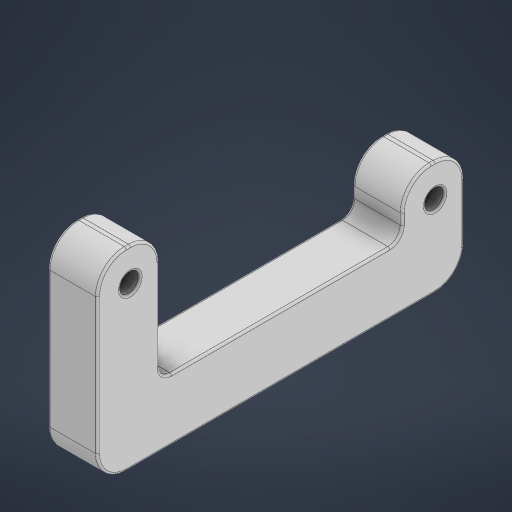
# Autodesk Inventor part: carb-holder
Saved by Autodesk Inventor 2024.2 (Build 282272000, 272)
## iProperties
Created: 2025-06-22
Part Number: carb-holder
Material: Generic
Document SubType Name: Modeling
Designer: Moe
Density: 1 g/cm^3
Appearance: Default
Author: Moe
Autodesk Inventor part; units mm, degrees
ref_plane "YZ Plane" through (0, 0, 0) normal (1, 0, 0) x (0, 1, 0)
ref_plane "XZ Plane" through (0, 0, 0) normal (0, 1, 0) x (-1, 0, 0)
ref_plane "XY Plane" through (0, 0, 0) normal (0, 0, 1) x (1, 0, 0)
sketch "Sketch1" plane through (0, 0, 0) normal (1, 0, 0) x (0, 1, 0)
  circle A0 centre (6.7632, 35.6186) radius 2.375
  circle A1 centre (-12.6339, -38.3814) radius 2.375
  line L0 (7.7632, 28.6186) -> (-14.2368, 28.6186)
  line L1 (-17.2368, 25.6186) -> (-17.2368, -27.3814)
  line L2 (-14.2368, -30.3814) -> (-11.6339, -30.3814)
  line L3 (-4.6339, -37.3814) -> (-4.6339, -38.3814)
  line L4 (-11.6339, -45.3814) -> (-25.2368, -45.3814)
  line L5 (-32.2368, -38.3814) -> (-32.2368, 36.6186)
  line L6 (-25.2368, 43.6186) -> (7.7632, 43.6186)
  line L7 (14.7632, 36.6186) -> (14.7632, 35.6186)
  arc A2 (-14.2368, 28.6186) -> (-17.2368, 25.6186) centre (-14.2368, 25.6186) ccw
  arc A3 (-17.2368, -27.3814) -> (-14.2368, -30.3814) centre (-14.2368, -27.3814) ccw
  arc A4 (14.7632, 36.6186) -> (7.7632, 43.6186) centre (7.7632, 36.6186) ccw
  arc A5 (7.7632, 28.6186) -> (14.7632, 35.6186) centre (7.7632, 35.6186) ccw
  arc A6 (-4.6339, -37.3814) -> (-11.6339, -30.3814) centre (-11.6339, -37.3814) ccw
  arc A7 (-11.6339, -45.3814) -> (-4.6339, -38.3814) centre (-11.6339, -38.3814) ccw
  arc A8 (-32.2368, -38.3814) -> (-25.2368, -45.3814) centre (-25.2368, -38.3814) ccw
  arc A9 (-25.2368, 43.6186) -> (-32.2368, 36.6186) centre (-25.2368, 36.6186) ccw
  point P0 (0, 0)
  point P1 (-4.6339, -37.8814)
  dimension "d0" = 76.5
  dimension "d1" = 4.75
  dimension "d2" = 4.75
  dimension "d3" = 59
  dimension "d4" = 7
  dimension "d5" = 8
  dimension "d6" = 15
  dimension "d7" = 15
  dimension "d9" = 8
  dimension "d10" = 8
  dimension "d11" = 24
  dimension "d12" = 15
  dimension "d13" = 3
  dimension "d14" = 7
  constraints: 16 end point, 16 point on circle, 16 tangent, 10 centre point, 7 perpendicular, 6 equal radius, 1 horizontal, 1 midpoint
  measures "d0" distance of A1.centre A0.centre
  measures "d1" diameter of A0
  measures "d2" diameter of A1
  measures "d3" distance between parallel lines of L2 L0
  measures "d4" distance from line of L0 A0.centre
  measures "d5" distance from line of L2 A1.centre
  measures "d6" distance between parallel lines of L6 L0
  measures "d7" distance between parallel lines of L4 L2
  measures "d9" distance from line of L7 A0.centre
  measures "d10" horizontal distance of point (-4.634, -37.881) A1.centre
  measures "d11" distance from line of L1 A0.centre
  measures "d12" distance between parallel lines of L1 L5
  measures "d13" radius of A2
  measures "d14" radius of A4
extrude "Extrusion1" add sketch "Sketch1" along normal blind 12
fillet "Fillet1" radius 0.5 32 edges at (12, -30.1865, 41.5683) (12, -32.2368, -0.8814) (12, -30.1865, -43.3312) (12, -18.4353, -45.3814) (12, -6.6842, -43.3312) (12, -4.6339, -37.8814) (12, -6.6842, -32.4317) (12, -12.9353, -30.3814) (12, -16.3581, -29.5027) (12, -17.2368, -0.8814) (12, -16.3581, 27.7399) (12, -3.2368, 28.6186) (12, 12.713, 30.6688) (12, 14.7632, 36.1186) (12, 12.713, 41.5683) (12, -8.7368, 43.6186) (0, -30.1865, 41.5683) (0, -32.2368, -0.8814) (0, -30.1865, -43.3312) (0, -18.4353, -45.3814) (0, -6.6842, -43.3312) (0, -4.6339, -37.8814) (0, -6.6842, -32.4317) (0, -12.9353, -30.3814) (0, -16.3581, -29.5027) (0, -17.2368, -0.8814) (0, -16.3581, 27.7399) (0, -3.2368, 28.6186) (0, 12.713, 30.6688) (0, 14.7632, 36.1186) (0, 12.713, 41.5683) (0, -8.7368, 43.6186)
fillet "Fillet2" radius 0.5 4 edges at (12, 4.3882, 35.6186) (0, -15.0089, -38.3814) (12, -15.0089, -38.3814) (0, 4.3882, 35.6186)
body "Solid1"
